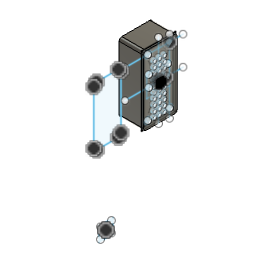
la+cosa (Autodesk Fusion 360 design; units mm, degrees)
Autodesk Fusion 360 part; units mm, degrees
sketch "main_shape" plane through (-3, 0, 0) normal (-1, 0, 0) x (0, -1, 0)
  line L0 (-16, -35.5) -> (16, -35.5)
  line L1 (16, -35.5) -> (16, 35.5)
  line L2 (16, 35.5) -> (-16, 35.5)
  line L3 (-16, 35.5) -> (-16, -35.5)
  line L4 (-16, -35.5) -> (16, 35.5) construction
  line L5 (16, -35.5) -> (-16, 35.5) construction
  line L6 (-12, -41.3396) -> (-12, 39)
  line L7 (37, 0) -> (-27, 0)
  line L8 (37, 31.5) -> (-27, 31.5)
  circle A0 centre (-12, 31.5) radius 1.5
  circle A1 centre (-12, -31.5) radius 1.5
  line L9 (0, 42) -> (0, -40.4906)
  circle A2 centre (12, 31.5) radius 1.5
  circle A3 centre (12, -31.5) radius 1.5
  line L10 (18.5, -38) -> (18.5, 38)
  line L11 (18.5, 38) -> (-18.5, 38)
  line L12 (-18.5, 38) -> (-18.5, -38)
  line L13 (-18.5, -38) -> (18.5, -38)
  spline S0 degree 3 poles (44.3606, -31.4828) (42.7106, -31.4828) (41.3606, -30.1328) (41.3606, -28.4828) knots 1 1 1 1 2 2 2 2
  circle A4 centre (67.7694, -28.0995) radius 1.4
  circle A5 centre (44.7721, -28.0995) radius 1.4
  line L14 (68.3606, -31.4828) -> (44.3606, -31.4828)
  spline S1 degree 3 poles (71.3606, -28.4828) (71.3606, -30.1328) (70.0106, -31.4828) (68.3606, -31.4828) knots 7 7 7 7 8 8 8 8
  line L15 (0.4061, -10.074) -> (-12.0849, -10.074)
  line L16 (41.3606, -28.4828) -> (41.3606, 30.5172)
  line L17 (71.3606, 30.5172) -> (71.3606, -28.4828)
  line L18 (-12.0849, 13.92) -> (12.9147, 13.92)
  line L19 (44.3606, 33.5172) -> (68.3606, 33.5172)
  line L20 (12.9147, -10.074) -> (0.4061, -10.074)
  line L21 (5.4993, -4.9973) -> (-5.0007, -4.9956)
  line L22 (-4.999, 5.5044) -> (5.501, 5.5027)
  line L23 (50.5, -120.5) -> (65.5, -120.5)
  line L24 (65.5, -120.5) -> (65.5, -105.5)
  circle A6 centre (-10.0913, 11.9264) radius 1.5
  line L25 (5.501, 5.5027) -> (5.4993, -4.9973)
  line L26 (5.501, 5.5027) -> (-5.0007, -4.9956) construction
  circle A7 centre (10.9961, 11.9264) radius 1.5
  circle A8 centre (58, -113) radius 4
  line L27 (5.4993, -4.9973) -> (-4.999, 5.5044) construction
  line L28 (-5.0007, -4.9956) -> (-4.999, 5.5044)
  spline S2 degree 3 poles (41.3606, 30.5172) (41.3606, 32.1672) (42.7106, 33.5172) (44.3606, 33.5172) knots 3 3 3 3 4 4 4 4
  line L29 (-12.0849, -10.074) -> (-12.0849, 13.92)
  circle A9 centre (67.7694, 29.8978) radius 1.4
  circle A10 centre (-10.0913, -0.5652) radius 1.5
  circle A11 centre (44.7718, 29.8978) radius 1.4
  line L30 (64.5, -119.5) -> (51.5, -119.5)
  spline S3 degree 3 poles (68.3606, 33.5172) (70.0106, 33.5172) (71.3606, 32.1672) (71.3606, 30.5172) knots 5 5 5 5 6 6 6 6
  line L31 (51.5, -119.5) -> (64.5, -106.5) construction
  line L32 (50.5, -105.5) -> (50.5, -120.5)
  line L33 (65.5, -105.5) -> (50.5, -105.5)
  line L34 (64.5, -119.5) -> (51.5, -106.5) construction
  line L35 (65.5, -120.5) -> (50.5, -105.5) construction
  line L36 (12.9147, 13.92) -> (12.9147, -10.074)
  line L37 (52, -119) -> (64, -107) construction
  line L38 (64, -119) -> (52, -107) construction
  line L39 (51.5, -119.5) -> (51.5, -106.5)
  line L40 (50.5, -120.5) -> (65.5, -105.5) construction
  line L41 (51.5, -106.5) -> (64.5, -106.5)
  line L42 (64.5, -106.5) -> (64.5, -119.5)
  circle A12 centre (10.9211, -0.5307) radius 1.5
  circle A13 centre (12, 31.5) radius 3.5
  circle A14 centre (-12, 31.5) radius 3.5
  circle A15 centre (12, -31.5) radius 3.5
  circle A16 centre (-12, -31.5) radius 3.5
  circle A17 centre (0.5, -1) radius 2
  circle A18 centre (-5, 23) radius 2
  circle A19 centre (0.5, 23) radius 2
  circle A20 centre (6, 23) radius 2
  circle A21 centre (-5, 17) radius 2
  circle A22 centre (0.5, 17) radius 2
  circle A23 centre (6, 17) radius 2
  circle A24 centre (-5, 11) radius 2
  circle A25 centre (0.5, 11) radius 2
  circle A26 centre (6, 11) radius 2
  circle A27 centre (-5, 5) radius 2
  circle A28 centre (0.5, 5) radius 2
  circle A29 centre (6, 5) radius 2
  circle A30 centre (-5, -1) radius 2
  circle A31 centre (6, -1) radius 2
  circle A32 centre (10.9961, 11.9264) radius 2.75
  circle A33 centre (-10.0913, 11.9264) radius 2.75
  circle A34 centre (-10.0913, -0.5652) radius 2.75
  circle A35 centre (10.9211, -0.5307) radius 2.75
  circle A36 centre (-5, -7) radius 2
  circle A37 centre (0.5, -7) radius 2
  circle A38 centre (6, -7) radius 2
  circle A39 centre (-5, -13) radius 2
  circle A40 centre (0.5, -13) radius 2
  circle A41 centre (6, -13) radius 2
  circle A42 centre (-5, -19) radius 2
  circle A43 centre (0.5, -19) radius 2
  circle A44 centre (6, -19) radius 2
  circle A45 centre (-5, -25) radius 2
  circle A46 centre (0.5, -25) radius 2
  circle A47 centre (6, -25) radius 2
  circle A48 centre (-5, -31) radius 2
  circle A49 centre (0.5, -31) radius 2
  circle A50 centre (6, -31) radius 2
  point P0 (-8, 0)
  point P1 (58, -113)
  point P2 (0.2502, 0.2536)
  point P3 (58, -113)
  point P4 (58, -113)
  dimension "d80" = 32
  dimension "d81" = 71
  dimension "d84" = 31.5
  dimension "d85" = 3
  dimension "d86" = 2.5
  dimension "d103" = 12
  dimension "d104" = 15
  dimension "d105" = 8
  dimension "d106" = 13
  dimension "d107" = 13
  dimension "d108" = 10.5
  dimension "d109" = 10.5
  dimension "d110" = 3
  dimension "d111" = 3
  dimension "d112" = 3
  dimension "d113" = 3
  dimension "d114" = 7
  dimension "d115" = 7
  dimension "d116" = 7
  dimension "d129" = 4
  dimension "d132" = 5.5
  dimension "d133" = -30
  dimension "d138" = 5.5
  dimension "d139" = 5.5
  dimension "d140" = 5.5
  dimension "d141" = 5.5
  constraint horizontal L0
  constraint perpendicular L0 L1
  constraint parallel L0 L2
  constraint parallel L1 L3
  constraint coincident L4 origin
  constraint coincident L5 origin
  constraint perpendicular L2 L6
  constraint horizontal L7
  constraint coincident L8 A0.centre
  constraint coincident L6 A0.centre
  constraint symmetric L7 A0 A1
  constraint perpendicular L8 L9
  constraint symmetric A0 L9 A2
  constraint symmetric A1 L9 A3
  constraint coincident L7 P0
  constraint coincident P4 L37
  constraint coincident P4 L38
  constraint horizontal L23
  constraint perpendicular L23 L24
  constraint parallel L23 L33
  constraint parallel L24 L32
  constraint coincident P4 L40
  constraint coincident P4 L35
  constraint coincident P4 P3
  constraint horizontal L30
  constraint perpendicular L30 L39
  constraint parallel L30 L41
  constraint parallel L39 L42
  constraint coincident P4 L34
  constraint coincident P4 L31
  constraint perpendicular L21 L25
  constraint parallel L25 L28
  constraint parallel L21 L22
  constraint coincident P2 L26
  constraint coincident P2 L27
  constraint concentric A2 A13
  constraint symmetric L9 A13 A14
  constraint concentric A3 A15
  constraint concentric A1 A16
  constraint concentric A7 A32
  constraint concentric A6 A33
  constraint concentric A10 A34
  constraint concentric A12 A35
  measures "d80" distance of L1.end L2.end
  measures "d81" distance of L0.end L1.end
  measures "d85" diameter of A0
  measures "d103" distance of L38.end L37.end
  measures "d104" distance of L24.end L32.start
  measures "d105" diameter of A8
  measures "d106" distance of L34.end L31.end
  measures "d107" distance of L30.end L34.end
  measures "d108" distance of L21.end L22.start
  measures "d109" distance of L21.start L21.end
  measures "d110" diameter of A6
  measures "d111" diameter of A10
  measures "d112" diameter of A12
  measures "d113" diameter of A7
  measures "d114" diameter of A13
  measures "d115" diameter of A15
  measures "d116" diameter of A16
  measures "d129" diameter of A17
  measures "d138" diameter of A32
  measures "d139" diameter of A33
  measures "d140" diameter of A34
  measures "d141" diameter of A35
extrude "Extrude23" add sketch "main_shape" against normal blind 2 contours L0 L3 L6 L7 L15 L29 A16 A34 | L0 L3 L6 L7 L12 L13 | L0 L6 L9 L15 A16 A40 A43 A46 A49 | L0 L6 L9 L13 | L3 L7 L8 L12 | L3 L6 L7 L8 L18 L29 A14 A33 A34 | L0 L1 L7 L9 L15 L20 L36 A35 A40 A43 A46 A49 | L0 L1 L7 L9 L10 L13 | L6 A1 A16 | L6 A1 A16 | L2 L3 L6 L8 L11 L12 | L2 L3 L6 L8 A14 | L7 L29 A34 | L7 L29 A34 | L9 A49 | L9 A49 | L6 A1 | L6 A1 | L6 L8 A0 A14 | L6 L8 A0 A14 | L6 L7 L29 A34 | L6 L7 L29 A34 | L6 L29 A33 A34 | L6 L15 L29 A34 | L1 L7 L8 L9 L18 L36 A13 A19 A22 A32 A35 | L1 L7 L8 L10 | L6 L7 L9 L15 L21 L28 A30 A34 A37 | L2 L6 L9 L11 | L2 L6 L8 L9 A14 | L6 L8 A0 | L6 L8 A0 | L6 L8 A0 A14 | L6 L8 L9 L18 A14 A19 A22 A33 | L6 L8 A0 A14 | L6 L7 A10 A34 | L6 L7 A10 A34 | L29 A33 | L6 L29 A33 | L6 L7 L9 L18 L22 L28 A25 A27 A28 A30 A33 A34 | L1 L2 L8 L9 A13 | L1 L2 L8 L9 L10 L11 | L7 L36 A35 | L7 L36 A35 | L9 A46 | L9 A46 | L7 L9 L15 L20 L21 L25 L36 A31 A35 A37 | L6 L8 A0 | L6 L8 A0 | L6 L18 A33 | L6 L18 L29 A33 | L7 A10 | L6 L18 A33 | L8 A2 A13 | L8 A2 A13 | L7 L36 A12 A35 | L7 L36 A12 A35 | L7 L9 L18 L22 L25 L36 A25 A28 A29 A31 A32 A35 | L9 A37 | L9 A37 | L9 A40 | L9 A40 | L18 A33 | L7 L28 A30 | L7 L28 A30 | L8 A2 | L8 A2 | L7 A12 | L18 L36 A32 | L36 A32 | L9 A43 | L9 A43 | L9 A19 | L9 A19 | L18 L36 A32 | L18 A32 | L7 L25 A31 | L7 L25 A31 | L22 L28 A27 | L9 A22 | L9 A22 | L9 A25 | L9 A25 | L22 L25 A29 | L9 L22 A28 | L9 L22 A28 | A3 | A15 | A18 | A20 | A21 | A23 | A24 | A26 | A36 | A38 | A39 | A41 | A42 | A44 | A45 | A47 | A48 | A50 picked at (-9.7033, 0.127) picked at (-5.0991, 0.6592) picked at (-5.0995, -1.9925) picked at (10.7507, 0.3866) picked at (6.4927, -1.8218) picked at (5.5949, 0.6416) picked at (-5.0979, 3.8421) picked at (7.1601, 5.2635) picked at (-0.5418, 6.1699) picked at (1.5934, 5.5934)
extrude "Extrude24" add sketch "main_shape" along normal blind 20 contours L0 L3 L6 L7 L12 L13 | L0 L6 L9 L13 | L3 L7 L8 L12 | L0 L1 L7 L9 L10 L13 | L2 L3 L6 L8 L11 L12 | L1 L7 L8 L10 | L2 L6 L9 L11 | L1 L2 L8 L9 L10 L11
extrude "Extrude25" add sketch "main_shape" along normal blind 8 contours L6 A1 A16 | L6 A1 A16 | L6 L8 A0 A14 | L6 L8 A0 A14 | L6 L8 A0 A14 | L6 L8 A0 A14 | L8 A2 A13 | L8 A2 A13 | A15
extrude "Extrude26" add sketch "main_shape" along normal blind 3 contours L0 L3 L6 L7 L15 L29 A16 A34 | L0 L6 L9 L15 A16 A40 A43 A46 A49 | L3 L6 L7 L8 L18 L29 A14 A33 A34 | L0 L1 L7 L9 L15 L20 L36 A35 A40 A43 A46 A49 | L2 L3 L6 L8 A14 | L7 L29 A34 | L7 L29 A34 | L9 A49 | L9 A49 | L1 L7 L8 L9 L18 L36 A13 A19 A22 A32 A35 | L2 L6 L8 L9 A14 | L6 L8 L9 L18 A14 A19 A22 A33 | L29 A33 | L1 L2 L8 L9 A13 | L7 L36 A35 | L7 L36 A35 | L9 A46 | L9 A46 | L9 A40 | L9 A40 | L18 A33 | L36 A32 | L9 A43 | L9 A43 | L9 A19 | L9 A19 | L18 A32 | L9 A22 | L9 A22 | A18 | A20 | A21 | A23 | A39 | A41 | A42 | A44 | A45 | A47 | A48 | A50
extrude "Extrude27" cut sketch "main_shape" against normal blind 14 contours L7 A10 | L7 A12 picked at (-9.7033, 0.127) picked at (10.7507, 0.3866)
extrude "Extrude28" cut sketch "main_shape" along normal mid plane 36 contours L9 A49 | L9 A49 | L9 A46 | L9 A46 | L9 A40 | L9 A40 | L9 A43 | L9 A43 | L9 A19 | L9 A19 | L9 A22 | L9 A22 | L9 A25 | L9 A25 | A18 | A20 | A21 | A23 | A24 | A26 | A39 | A41 | A42 | A44 | A45 | A47 | A48 | A50
extrude "Extrude29" add 1 faces at (-23, -17.6667, -11.8333) along direction (-1, 0, 0) blind 5
extrude "Extrude30" add sketch "main_shape" along normal blind 2 contours L7 L29 A34 | L7 L29 A34 | L6 L7 L29 A34 | L6 L7 L29 A34 | L6 L7 A10 A34 | L6 L7 A10 A34 | L29 A33 | L7 L36 A35 | L7 L36 A35 | L6 L18 A33 | L7 L36 A12 A35 | L7 L36 A12 A35 | L18 A33 | L18 L36 A32 | L36 A32 | L18 A32 picked at (-10.0539, 13.754) picked at (11.0335, 13.754)
fillet "Fillet9" radius 3 1 edges at (-14.5, -18.5, -38)
fillet "Fillet10" radius 3 1 edges at (-14.5, 18.5, -38)
fillet "Fillet11" radius 3 2 edges at (-14.5, -18.5, 38) (-14.5, 18.5, 38)
equation "d84 = ( 63 / 2 ) * 1 mm"
named bodies: "BottomCase"
